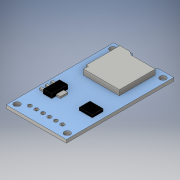
# Autodesk Inventor part: MicroSD Card Reader
Saved by Autodesk Inventor 2016 (Build 200138000, 138)
## iProperties
Created: 2015-11-27
Part Number: MicroSD Card Reader
Material: Generic
Document SubType Name: Modeling
Designer: Spooner
Density: 1 g/cm^3
Appearance: Default
Author: Spooner
Autodesk Inventor part; units mm, degrees
ref_plane "YZ Plane" through (0, 0, 0) normal (1, 0, 0) x (0, 1, 0)
ref_plane "XZ Plane" through (0, 0, 0) normal (0, 1, 0) x (-1, 0, 0)
ref_plane "XY Plane" through (0, 0, 0) normal (0, 0, 1) x (1, 0, 0)
sketch "Sketch1" plane through (0, 0, 0) normal (0, 1, 0) x (-1, 0, 0)
  line L0 (0, 0) -> (-23.5077, 0)
  line L1 (-23.5077, 0) -> (-23.5077, -41.9735)
  line L2 (0, -41.9735) -> (0, 0)
  line L3 (-7.4041, -41.9735) -> (-8.8011, -40.5765)
  line L4 (-8.8011, -40.5765) -> (-16.3322, -40.5765)
  line L5 (-16.3322, -40.5765) -> (-17.7292, -41.9735)
  line L6 (-23.5077, -41.9735) -> (-17.7292, -41.9735)
  line L7 (-7.4041, -41.9735) -> (0, -41.9735)
  circle A0 centre (-1.9431, -39.6748) radius 1.1811
  circle A1 centre (-21.5646, -39.6748) radius 1.1811
  circle A2 centre (-21.5646, -2.2987) radius 1.1811
  circle A3 centre (-1.9431, -2.2987) radius 1.1811
  dimension "d0" = 135
  dimension "d1" = 41.9735
  dimension "d2" = 23.5077
  dimension "d3" = 1.397
  dimension "d4" = 5.7785
  dimension "d5" = 7.4041
  dimension "d6" = 2.3622
  dimension "d7" = 1.1176
  dimension "d8" = 0.762
  dimension "d9" = 0.762
  dimension "d10" = 1.1176
  constraints: 16 end point, 4 centre point, 3 equal radius, 3 horizontal alignment, 3 parallel, 2 horizontal, 2 perpendicular, 2 vertical alignment
  measures "d0" angle of L4 L3
  measures "d1" distance of L2.start L0.start
  measures "d2" distance of L0.start L0.end
  measures "d3" distance between parallel lines of L4 L6
  measures "d4" distance of L1.end L5.end
  measures "d5" distance of L3.start L2.start
  measures "d6" diameter of A0
  measures "d7" distance edge to line of A1 L6
  measures "d8" distance edge to line of A1 L1
  measures "d9" distance edge to line of A0 L2
  measures "d10" distance edge to line of A2 L0
extrude "Extrusion1" add sketch "Sketch1" along normal blind 1.2446
sketch "Sketch2" plane through (0, 1.2446, 0) normal (0, 1, 0) x (1, 0, 0)
  line L0 (9.7028, 39.1795) -> (19.0627, 39.1795)
  line L1 (19.0627, 39.1795) -> (19.0627, 25.146)
  line L2 (19.0627, 25.146) -> (5.08, 25.146)
  line L3 (4.2418, 26.9875) -> (4.2418, 40.1955)
  line L4 (4.2418, 40.1955) -> (8.0518, 40.1955)
  line L5 (8.0518, 40.1955) -> (9.7028, 39.1795)
  line L6 (5.08, 25.146) -> (5.08, 26.9875)
  line L7 (16.3322, 40.5765) -> (8.8011, 40.5765) projected
  line L8 (0, 41.9735) -> (0, 0) projected
  line L9 (4.2418, 26.9875) -> (5.08, 26.9875)
  line L10 (7.4041, 41.9735) -> (0, 41.9735) projected
  point P0 (4.6609, 26.9875)
  dimension "d13" = 14.0335
  dimension "d14" = 1.397
  dimension "d15" = 14.8209
  dimension "d16" = 4.2418
  dimension "d17" = 5.08
  dimension "d18" = 13.208
  dimension "d20" = 1.778
  dimension "d21" = 9.3599
  dimension "d22" = 3.81
  constraints: 16 end point, 2 horizontal, 2 perpendicular, 1 horizontal alignment, 1 midpoint, 1 parallel, 1 vertical
  measures "d13" distance between parallel lines of L2 L0
  measures "d14" distance between parallel lines of L0 L7
  measures "d15" distance between parallel lines of L1 L3
  measures "d16" distance between parallel lines of L8 L3
  measures "d17" distance between parallel lines of L8 L6
  measures "d18" distance of L3.start L3.end
  measures "d20" distance between parallel lines of L4 L10
  measures "d21" distance from line of L0.start L1
  measures "d22" distance of L3.end L4.end
extrude "Extrusion2" add sketch "Sketch2" along normal blind 2.032
sketch "Sketch3" plane through (8.0518, 1.2446, -40.1955) normal (0, 0, -1) x (-1, 0, 0)
  line L0 (-10.1473, 1.778) -> (1.143, 1.778)
  line L1 (1.143, 1.778) -> (1.143, 1.0414)
  line L2 (1.143, 1.0414) -> (-10.1473, 1.0414)
  line L3 (-10.1473, 1.0414) -> (-10.1473, 1.778)
  line L4 (2.9718, 2.032) -> (-11.0109, 2.032) projected
  line L5 (-8.2804, -1.2446) -> (-0.7493, -1.2446) projected
  line L6 (-11.0109, 0) -> (-11.0109, 2.032) projected
  line L7 (3.81, 0) -> (3.81, 2.032) projected
  point P0 (8.0518, -1.2446)
  dimension "d25" = 0.254
  dimension "d26" = 2.286
  dimension "d27" = 0.8636
  dimension "d28" = 2.667
  constraints: 8 end point, 2 parallel, 1 horizontal, 1 perpendicular
  measures "d25" distance between parallel lines of L4 L0
  measures "d26" distance between parallel lines of L5 L2
  measures "d27" distance from line of L6 L0.start
  measures "d28" distance between parallel lines of L7 L1
extrude "Extrusion3" cut sketch "Sketch3" against normal blind 12.192
sketch "Sketch4" plane through (0, 1.2446, 0) normal (0, 1, 0) x (1, 0, 0)
  line L0 (3.5179, 10.9474) -> (6.8199, 10.9474)
  line L1 (6.8199, 10.9474) -> (6.8199, 17.3228)
  line L2 (6.8199, 17.3228) -> (3.5179, 17.3228)
  line L3 (3.5179, 17.3228) -> (3.5179, 10.9474)
  line L4 (5.08, 25.146) -> (19.0627, 25.146) projected
  line L5 (0, 41.9735) -> (0, 0) projected
  dimension "d31" = 6.3754
  dimension "d32" = 3.302
  dimension "d33" = 7.8232
  dimension "d34" = 3.5179
  constraints: 8 end point, 2 parallel, 1 horizontal, 1 perpendicular
  measures "d31" distance of L2.end L0.start
  measures "d32" distance of L1.end L2.end
  measures "d33" distance between parallel lines of L4 L2
  measures "d34" distance between parallel lines of L5 L3
extrude "Extrusion4" add sketch "Sketch4" along normal blind 1.6002
sketch "Sketch5" plane through (0, 1.2446, 0) normal (0, 1, 0) x (1, 0, 0)
  line L0 (3.5179, 10.9474) -> (3.5179, 17.3228) projected
  line L1 (1.4859, 16.764) -> (3.5179, 16.764)
  line L2 (3.5179, 16.764) -> (3.5179, 15.875)
  line L3 (3.5179, 15.875) -> (1.4859, 15.875)
  line L4 (1.4859, 15.875) -> (1.4859, 16.764)
  line L5 (1.4859, 14.5796) -> (3.5179, 14.5796)
  line L6 (3.5179, 14.5796) -> (3.5179, 13.6906)
  line L7 (3.5179, 13.6906) -> (1.4859, 13.6906)
  line L8 (1.4859, 13.6906) -> (1.4859, 14.5796)
  line L9 (1.4859, 12.3952) -> (3.5179, 12.3952)
  line L10 (3.5179, 12.3952) -> (3.5179, 11.5062)
  line L11 (3.5179, 11.5062) -> (1.4859, 11.5062)
  line L12 (1.4859, 11.5062) -> (1.4859, 12.3952)
  line L13 (3.5179, 17.3228) -> (3.5179, 10.9474) projected
  line L14 (6.8199, 17.3228) -> (6.8199, 10.9474) projected
  line L15 (6.8199, 15.5765) -> (8.4709, 15.5765)
  line L16 (8.4709, 15.5765) -> (8.4709, 12.6936)
  line L17 (8.4709, 12.6936) -> (6.8199, 12.6936)
  line L18 (6.8199, 12.6936) -> (6.8199, 15.5765)
  point P0 (0, 0)
  point P1 (1.4859, 14.1351)
  point P2 (3.5179, 14.1351)
  point P3 (8.4709, 14.1351)
  dimension "d37" = 0.889
  dimension "d38" = 2.032
  dimension "d39" = 5.2578
  dimension "d40" = 1.2954
  dimension "d41" = 1.2954
  dimension "d44" = 2.8829
  dimension "d45" = 1.651
  constraints: 32 end point, 8 parallel, 6 point on line, 4 horizontal, 4 perpendicular, 3 midpoint, 2 collinear, 2 horizontal alignment
  measures "d37" distance of L3.end L1.start
  measures "d38" distance of point (3.518, 14.135) point (1.486, 14.135)
  measures "d39" distance between parallel lines of L11 L1
  measures "d40" distance between parallel lines of L5 L3
  measures "d41" distance between parallel lines of L9 L7
  measures "d44" distance of L15.end L16.end
  measures "d45" distance from line of L14 point (8.471, 14.135)
extrude "Extrusion5" add sketch "Sketch5" along normal blind 0.635
sketch "Sketch6" plane through (0, 1.2446, 0) normal (0, 1, 0) x (1, 0, 0)
  line L0 (16.129, 16.637) -> (21.2598, 16.637)
  line L1 (21.2598, 16.637) -> (21.2598, 12.3698)
  line L2 (21.2598, 12.3698) -> (16.129, 12.3698)
  line L3 (16.129, 12.3698) -> (16.129, 16.637)
  line L4 (23.5077, 0) -> (23.5077, 41.9735) projected
  line L5 (5.08, 25.146) -> (19.0627, 25.146) projected
  point P0 (0, 0)
  dimension "d46" = 5.1308
  dimension "d47" = 4.2672
  dimension "d48" = 2.2479
  dimension "d49" = 8.509
  constraints: 8 end point, 2 parallel, 1 horizontal, 1 perpendicular
  measures "d46" distance of L0.start L0.end
  measures "d47" distance of L0.end L1.end
  measures "d48" distance between parallel lines of L4 L1
  measures "d49" distance between parallel lines of L5 L0
extrude "Extrusion6" add sketch "Sketch6" along normal blind 1.016
sketch "Sketch7" plane through (0, 1.2446, 0) normal (0, 1, 0) x (1, 0, 0)
  circle A0 centre (4.953, 4.318) radius 0.508
  line L0 (0, 0) -> (23.5077, 0) projected
  line L1 (0, 41.9735) -> (0, 0) projected
  dimension "d52" = 1.016
  dimension "d53" = 3.81
  dimension "d54" = 4.445
  constraints: 1 centre point
  measures "d52" diameter of A0
  measures "d53" distance edge to line of A0 L0
  measures "d54" distance edge to line of A0 L1
extrude "Extrusion7" cut sketch "Sketch7" against normal through all
sketch "Sketch8" plane through (0, 1.2446, 0) normal (0, 1, 0) x (1, 0, 0)
  circle A0 centre (4.953, 4.318) radius 0.762
  circle A1 centre (4.953, 4.318) radius 0.508 projected
  point P0 (0, 0)
  dimension "d57" = 1.524
  constraints: 1 centre point, 1 concentric
  measures "d57" diameter of A0
extrude "Extrusion8" add sketch "Sketch8" along normal blind 0.0254
pattern_linear "Rectangular Pattern1" count 6 spacing 2.54 along (1, 0, 0) of "Extrusion7", "Extrusion8"
sketch "Sketch9" plane through (0, 0, 0) normal (0, -1, 0) x (1, 0, 0)
  line L0 (18.4451, -5.588) -> (18.4451, -7.6539) construction
  line L1 (18.4451, -7.6539) -> (16.8609, -7.6539) construction
  line L2 (16.8609, -7.6539) -> (16.8609, -5.588) construction
  line L3 (16.8609, -5.588) -> (18.4451, -5.588) construction
  circle A0 centre (17.653, -4.318) radius 0.508 projected
  circle A1 centre (15.113, -4.318) radius 0.508 projected
  circle A2 centre (12.573, -4.318) radius 0.508 projected
  circle A3 centre (10.033, -4.318) radius 0.508 projected
  circle A4 centre (7.493, -4.318) radius 0.508 projected
  circle A5 centre (4.953, -4.318) radius 0.508 projected
  line L4 (13.825, -5.588) -> (13.825, -7.6539) construction
  line L5 (13.825, -7.6539) -> (16.401, -7.6539) construction
  line L6 (16.401, -7.6539) -> (16.401, -5.588) construction
  line L7 (16.401, -5.588) -> (13.825, -5.588) construction
  line L8 (13.5877, -5.588) -> (13.5877, -7.6539) construction
  line L9 (13.5877, -7.6539) -> (11.5583, -7.6539) construction
  line L10 (11.5583, -7.6539) -> (11.5583, -5.588) construction
  line L11 (11.5583, -5.588) -> (13.5877, -5.588) construction
  line L12 (10.3041, -5.588) -> (10.3041, -7.6539) construction
  line L13 (10.3041, -7.6539) -> (9.7619, -7.6539) construction
  line L14 (9.7619, -7.6539) -> (9.7619, -5.588) construction
  line L15 (9.7619, -5.588) -> (10.3041, -5.588) construction
  line L16 (7.9729, -5.588) -> (7.9729, -7.6539) construction
  line L17 (7.9729, -7.6539) -> (7.0131, -7.6539) construction
  line L18 (7.0131, -7.6539) -> (7.0131, -5.588) construction
  line L19 (7.0131, -5.588) -> (7.9729, -5.588) construction
  line L20 (5.7817, -5.588) -> (5.7817, -7.6539) construction
  line L21 (5.7817, -7.6539) -> (4.1243, -7.6539) construction
  line L22 (4.1243, -7.6539) -> (4.1243, -5.588) construction
  line L23 (4.1243, -5.588) -> (5.7817, -5.588) construction
  spline S0 degree 2 poles (17.2026, -6.5593) (17.0886, -6.4666) (17.0006, -6.2897) (17.0006, -6.165) knots 0 0 0 1 2 2 2
  spline S1 degree 2 poles (17.0006, -6.165) (17.0006, -5.9524) (17.1804, -5.818) knots 0 0 0 1 1 1
  spline S2 degree 2 poles (17.1804, -5.818) (17.3621, -5.6798) (17.6559, -5.6798) knots 0 0 0 1 1 1
  spline S3 degree 2 poles (17.6559, -5.6798) (17.9806, -5.6798) (18.1508, -5.8354) knots 0 0 0 1 1 1
  spline S4 degree 2 poles (18.1508, -5.8354) (18.287, -5.9601) (18.287, -6.1399) knots 0 0 0 1 1 1
  spline S5 degree 2 poles (18.287, -6.1399) (18.287, -6.28) (18.2455, -6.3612) knots 0 0 0 1 1 1
  spline S6 degree 2 poles (18.2455, -6.3612) (18.1991, -6.4511) (18.0841, -6.5139) knots 0 0 0 1 1 1
  spline S7 degree 2 poles (18.0841, -6.5139) (18.0599, -6.5275) (18.0377, -6.5275) knots 0 0 0 1 1 1
  spline S8 degree 2 poles (18.0377, -6.5275) (17.999, -6.5275) (17.9459, -6.4695) (17.9459, -6.4337) knots 0 0 0 1 2 2 2
  spline S9 degree 2 poles (17.9459, -6.4337) (17.9459, -6.3834) (18, -6.3544) knots 0 0 0 1 1 1
  spline S10 degree 2 poles (18, -6.3544) (18.056, -6.3216) (18.0802, -6.2655) knots 0 0 0 1 1 1
  spline S11 degree 2 poles (18.0802, -6.2655) (18.1005, -6.223) (18.1005, -6.1389) knots 0 0 0 1 1 1
  spline S12 degree 2 poles (18.1005, -6.1389) (18.1005, -6.0297) (18.0029, -5.9543) knots 0 0 0 1 1 1
  spline S13 degree 2 poles (18.0029, -5.9543) (17.885, -5.8615) (17.6559, -5.8615) knots 0 0 0 1 1 1
  spline S14 degree 2 poles (17.6559, -5.8615) (17.4452, -5.8615) (17.1871, -6.0365) (17.1871, -6.1679) knots 0 0 0 1 2 2 2
  spline S15 degree 2 poles (17.1871, -6.1679) (17.1871, -6.31) (17.3225, -6.4173) knots 0 0 0 1 1 1
  spline S16 degree 2 poles (17.3225, -6.4173) (17.3553, -6.4443) (17.3553, -6.4859) knots 0 0 0 1 1 1
  spline S17 degree 2 poles (17.3553, -6.4859) (17.3553, -6.5217) (17.2983, -6.5816) (17.2606, -6.5816) knots 0 0 0 1 2 2 2
  spline S18 degree 2 poles (17.2606, -6.5816) (17.2297, -6.5816) (17.2026, -6.5593) knots 0 0 0 1 1 1
  spline S19 degree 2 poles (17.3669, -7.6718) (17.0006, -7.6718) (17.0006, -7.2195) knots 0 0 0 1 1 1
  spline S20 degree 2 poles (17.0006, -7.2195) (17.0006, -6.9479) (17.2722, -6.801) knots 0 0 0 1 1 1
  spline S21 degree 2 poles (17.2722, -6.801) (17.2896, -6.7903) (17.3167, -6.7903) knots 0 0 0 1 1 1
  spline S22 degree 2 poles (17.3167, -6.7903) (17.3572, -6.7903) (17.4201, -6.8503) (17.4201, -6.8889) knots 0 0 0 1 2 2 2
  spline S23 degree 2 poles (17.4201, -6.8889) (17.4201, -6.9353) (17.3775, -6.9537) knots 0 0 0 1 1 1
  spline S24 degree 2 poles (17.3775, -6.9537) (17.1871, -7.0397) (17.1871, -7.2195) knots 0 0 0 1 1 1
  spline S25 degree 2 poles (17.1871, -7.2195) (17.1871, -7.4843) (17.365, -7.4843) knots 0 0 0 1 1 1
  spline S26 degree 2 poles (17.365, -7.4843) (17.4529, -7.4843) (17.5225, -7.3181) knots 0 0 0 1 1 1
  spline S27 degree 2 poles (17.5225, -7.3181) (17.6569, -6.9972) (17.6598, -6.9904) knots 0 0 0 1 1 1
  spline S28 degree 2 poles (17.6598, -6.9904) (17.7728, -6.801) (17.9594, -6.801) knots 0 0 0 1 1 1
  spline S29 degree 2 poles (17.9594, -6.801) (18.1334, -6.801) (18.2232, -6.9286) knots 0 0 0 1 1 1
  spline S30 degree 2 poles (18.2232, -6.9286) (18.2938, -7.03) (18.2996, -7.1934) knots 0 0 0 1 1 1
  spline S31 degree 2 poles (18.2996, -7.1934) (18.3054, -7.3442) (18.2271, -7.4659) knots 0 0 0 1 1 1
  spline S32 degree 2 poles (18.2271, -7.4659) (18.1633, -7.5781) (18.0319, -7.6196) knots 0 0 0 1 1 1
  spline S33 degree 2 poles (18.0319, -7.6196) (18.0106, -7.6254) (17.9961, -7.6254) knots 0 0 0 1 1 1
  spline S34 degree 2 poles (17.9961, -7.6254) (17.9575, -7.6254) (17.9101, -7.5684) (17.9101, -7.5317) knots 0 0 0 1 2 2 2
  spline S35 degree 2 poles (17.9101, -7.5317) (17.9101, -7.464) (17.9623, -7.4476) knots 0 0 0 1 1 1
  spline S36 degree 2 poles (17.9623, -7.4476) (18.0415, -7.4224) (18.1208, -7.2842) (18.1169, -7.2001) knots 0 0 0 1 2 2 2
  spline S37 degree 2 poles (18.1169, -7.2001) (18.1082, -6.9827) (17.9633, -6.9827) knots 0 0 0 1 1 1
  spline S38 degree 2 poles (17.9633, -6.9827) (17.8869, -6.9827) (17.8337, -7.059) knots 0 0 0 1 1 1
  spline S39 degree 2 poles (17.8337, -7.059) (17.7931, -7.1161) (17.7439, -7.2523) knots 0 0 0 1 1 1
  spline S40 degree 2 poles (17.7439, -7.2523) (17.6694, -7.4592) (17.6201, -7.5307) knots 0 0 0 1 1 1
  spline S41 degree 2 poles (17.6201, -7.5307) (17.5225, -7.6718) (17.3669, -7.6718) knots 0 0 0 1 1 1
  spline S42 degree 2 poles (14.8269, -6.5439) (14.4606, -6.5439) (14.4606, -6.0916) knots 0 0 0 1 1 1
  spline S43 degree 2 poles (14.4606, -6.0916) (14.4606, -5.82) (14.7322, -5.6731) knots 0 0 0 1 1 1
  spline S44 degree 2 poles (14.7322, -5.6731) (14.7496, -5.6624) (14.7767, -5.6624) knots 0 0 0 1 1 1
  spline S45 degree 2 poles (14.7767, -5.6624) (14.8172, -5.6624) (14.8801, -5.7223) (14.8801, -5.761) knots 0 0 0 1 2 2 2
  spline S46 degree 2 poles (14.8801, -5.761) (14.8801, -5.8074) (14.8375, -5.8258) knots 0 0 0 1 1 1
  spline S47 degree 2 poles (14.8375, -5.8258) (14.6471, -5.9118) (14.6471, -6.0916) knots 0 0 0 1 1 1
  spline S48 degree 2 poles (14.6471, -6.0916) (14.6471, -6.3564) (14.825, -6.3564) knots 0 0 0 1 1 1
  spline S49 degree 2 poles (14.825, -6.3564) (14.9129, -6.3564) (14.9825, -6.1901) knots 0 0 0 1 1 1
  spline S50 degree 2 poles (14.9825, -6.1901) (15.1169, -5.8693) (15.1198, -5.8625) knots 0 0 0 1 1 1
  spline S51 degree 2 poles (15.1198, -5.8625) (15.2328, -5.6731) (15.4194, -5.6731) knots 0 0 0 1 1 1
  spline S52 degree 2 poles (15.4194, -5.6731) (15.5934, -5.6731) (15.6832, -5.8006) knots 0 0 0 1 1 1
  spline S53 degree 2 poles (15.6832, -5.8006) (15.7538, -5.9021) (15.7596, -6.0655) knots 0 0 0 1 1 1
  spline S54 degree 2 poles (15.7596, -6.0655) (15.7654, -6.2162) (15.6871, -6.338) knots 0 0 0 1 1 1
  spline S55 degree 2 poles (15.6871, -6.338) (15.6233, -6.4501) (15.4919, -6.4917) knots 0 0 0 1 1 1
  spline S56 degree 2 poles (15.4919, -6.4917) (15.4706, -6.4975) (15.4561, -6.4975) knots 0 0 0 1 1 1
  spline S57 degree 2 poles (15.4561, -6.4975) (15.4175, -6.4975) (15.3701, -6.4405) (15.3701, -6.4037) knots 0 0 0 1 2 2 2
  spline S58 degree 2 poles (15.3701, -6.4037) (15.3701, -6.3361) (15.4223, -6.3197) knots 0 0 0 1 1 1
  spline S59 degree 2 poles (15.4223, -6.3197) (15.5015, -6.2945) (15.5808, -6.1563) (15.5769, -6.0722) knots 0 0 0 1 2 2 2
  spline S60 degree 2 poles (15.5769, -6.0722) (15.5682, -5.8548) (15.4233, -5.8548) knots 0 0 0 1 1 1
  spline S61 degree 2 poles (15.4233, -5.8548) (15.3469, -5.8548) (15.2937, -5.9311) knots 0 0 0 1 1 1
  spline S62 degree 2 poles (15.2937, -5.9311) (15.2531, -5.9881) (15.2039, -6.1244) knots 0 0 0 1 1 1
  spline S63 degree 2 poles (15.2039, -6.1244) (15.1294, -6.3312) (15.0801, -6.4028) knots 0 0 0 1 1 1
  spline S64 degree 2 poles (15.0801, -6.4028) (14.9825, -6.5439) (14.8269, -6.5439) knots 0 0 0 1 1 1
  spline S65 degree 2 poles (14.6626, -7.6196) (14.5486, -7.5268) (14.4606, -7.35) (14.4606, -7.2253) knots 0 0 0 1 2 2 2
  spline S66 degree 2 poles (14.4606, -7.2253) (14.4606, -7.0126) (14.6404, -6.8783) knots 0 0 0 1 1 1
  spline S67 degree 2 poles (14.6404, -6.8783) (14.8221, -6.7401) (15.1159, -6.7401) knots 0 0 0 1 1 1
  spline S68 degree 2 poles (15.1159, -6.7401) (15.4406, -6.7401) (15.6108, -6.8957) knots 0 0 0 1 1 1
  spline S69 degree 2 poles (15.6108, -6.8957) (15.747, -7.0204) (15.747, -7.2001) knots 0 0 0 1 1 1
  spline S70 degree 2 poles (15.747, -7.2001) (15.747, -7.3403) (15.7055, -7.4215) knots 0 0 0 1 1 1
  spline S71 degree 2 poles (15.7055, -7.4215) (15.6591, -7.5114) (15.5441, -7.5742) knots 0 0 0 1 1 1
  spline S72 degree 2 poles (15.5441, -7.5742) (15.5199, -7.5877) (15.4977, -7.5877) knots 0 0 0 1 1 1
  spline S73 degree 2 poles (15.4977, -7.5877) (15.459, -7.5877) (15.4059, -7.5297) (15.4059, -7.494) knots 0 0 0 1 2 2 2
  spline S74 degree 2 poles (15.4059, -7.494) (15.4059, -7.4437) (15.46, -7.4147) knots 0 0 0 1 1 1
  spline S75 degree 2 poles (15.46, -7.4147) (15.516, -7.3819) (15.5402, -7.3258) knots 0 0 0 1 1 1
  spline S76 degree 2 poles (15.5402, -7.3258) (15.5605, -7.2833) (15.5605, -7.1992) knots 0 0 0 1 1 1
  spline S77 degree 2 poles (15.5605, -7.1992) (15.5605, -7.09) (15.4629, -7.0146) knots 0 0 0 1 1 1
  spline S78 degree 2 poles (15.4629, -7.0146) (15.345, -6.9218) (15.1159, -6.9218) knots 0 0 0 1 1 1
  spline S79 degree 2 poles (15.1159, -6.9218) (14.9052, -6.9218) (14.6471, -7.0967) (14.6471, -7.2282) knots 0 0 0 1 2 2 2
  spline S80 degree 2 poles (14.6471, -7.2282) (14.6471, -7.3703) (14.7825, -7.4775) knots 0 0 0 1 1 1
  spline S81 degree 2 poles (14.7825, -7.4775) (14.8153, -7.5046) (14.8153, -7.5462) knots 0 0 0 1 1 1
  spline S82 degree 2 poles (14.8153, -7.5462) (14.8153, -7.5819) (14.7583, -7.6418) (14.7206, -7.6418) knots 0 0 0 1 2 2 2
  spline S83 degree 2 poles (14.7206, -7.6418) (14.6897, -7.6418) (14.6626, -7.6196) knots 0 0 0 1 1 1
  spline S84 degree 2 poles (14.5969, -8.7253) (14.5882, -8.7359) (14.565, -8.7359) knots 0 0 0 1 1 1
  spline S85 degree 2 poles (14.565, -8.7359) (14.5263, -8.7359) (14.4712, -8.676) (14.4712, -8.6403) knots 0 0 0 1 2 2 2
  spline S86 degree 2 poles (14.4712, -8.6403) (14.4712, -8.5919) (14.5215, -8.5629) knots 0 0 0 1 1 1
  line L24 (14.5215, -8.5629) -> (15.1903, -8.1879)
  line L25 (15.1903, -8.1879) -> (15.0473, -8.0555)
  line L26 (15.0473, -8.0555) -> (14.565, -8.0555)
  spline S87 degree 2 poles (14.565, -8.0555) (14.4712, -8.0555) (14.4712, -7.9656) knots 0 0 0 1 1 1
  spline S88 degree 2 poles (14.4712, -7.9656) (14.4712, -7.8738) (14.565, -7.8738) knots 0 0 0 1 1 1
  line L27 (14.565, -7.8738) -> (15.6417, -7.8738)
  spline S89 degree 2 poles (15.6417, -7.8738) (15.7345, -7.8738) (15.7345, -7.9656) knots 0 0 0 1 1 1
  spline S90 degree 2 poles (15.7345, -7.9656) (15.7345, -8.0555) (15.6417, -8.0555) knots 0 0 0 1 1 1
  line L28 (15.6417, -8.0555) -> (15.2744, -8.0555)
  line L29 (15.2744, -8.0555) -> (15.7074, -8.4924)
  spline S91 degree 2 poles (15.7074, -8.4924) (15.7345, -8.5194) (15.7345, -8.5542) knots 0 0 0 1 1 1
  spline S92 degree 2 poles (15.7345, -8.5542) (15.7345, -8.591) (15.6765, -8.6461) (15.6407, -8.6461) knots 0 0 0 1 2 2 2
  spline S93 degree 2 poles (15.6407, -8.6461) (15.6021, -8.6461) (15.5905, -8.62) knots 0 0 0 1 1 1
  line L30 (15.5905, -8.62) -> (15.3073, -8.3145)
  line L31 (15.3073, -8.3145) -> (14.5969, -8.7253)
  spline S94 degree 2 poles (12.0231, -6.7198) (11.9293, -6.7198) (11.9293, -6.628) knots 0 0 0 1 1 1
  spline S95 degree 2 poles (11.9293, -6.628) (11.9293, -6.5362) (12.0231, -6.5362) knots 0 0 0 1 1 1
  line L32 (12.0231, -6.5362) -> (12.8765, -6.5362)
  line L33 (12.8765, -6.5362) -> (12.4947, -6.3023)
  spline S96 degree 2 poles (12.4947, -6.3023) (12.4358, -6.2607) (12.4358, -6.2008) knots 0 0 0 1 1 1
  spline S97 degree 2 poles (12.4358, -6.2008) (12.4358, -6.1428) (12.4899, -6.107) knots 0 0 0 1 1 1
  line L34 (12.4899, -6.107) -> (12.8852, -5.8751)
  line L35 (12.8852, -5.8751) -> (12.0231, -5.8751)
  spline S98 degree 2 poles (12.0231, -5.8751) (11.9293, -5.8751) (11.9293, -5.7832) knots 0 0 0 1 1 1
  spline S99 degree 2 poles (11.9293, -5.7832) (11.9293, -5.6895) (12.0231, -5.6895) knots 0 0 0 1 1 1
  line L36 (12.0231, -5.6895) -> (13.092, -5.6895)
  spline S100 degree 2 poles (13.092, -5.6895) (13.1906, -5.6895) (13.1906, -5.789) knots 0 0 0 1 1 1
  spline S101 degree 2 poles (13.1906, -5.789) (13.1906, -5.8577) (13.1355, -5.8963) knots 0 0 0 1 1 1
  line L37 (13.1355, -5.8963) -> (12.6774, -6.2037)
  line L38 (12.6774, -6.2037) -> (13.1258, -6.5072)
  spline S102 degree 2 poles (13.1258, -6.5072) (13.1993, -6.5584) (13.1993, -6.6241) knots 0 0 0 1 1 1
  spline S103 degree 2 poles (13.1993, -6.6241) (13.1993, -6.6647) (13.1374, -6.7198) (13.092, -6.7198) knots 0 0 0 1 2 2 2
  line L39 (13.092, -6.7198) -> (12.0231, -6.7198)
  spline S104 degree 2 poles (12.5585, -7.9511) (12.3033, -7.9511) (12.1371, -7.8313) knots 0 0 0 1 1 1
  spline S105 degree 2 poles (12.1371, -7.8313) (11.9206, -7.6911) (11.9206, -7.4756) knots 0 0 0 1 1 1
  spline S106 degree 2 poles (11.9206, -7.4756) (11.9206, -7.2591) (12.1207, -7.1209) knots 0 0 0 1 1 1
  spline S107 degree 2 poles (12.1207, -7.1209) (12.3043, -6.9923) (12.5585, -6.9923) knots 0 0 0 1 1 1
  spline S108 degree 2 poles (12.5585, -6.9923) (12.8127, -6.9923) (12.9992, -7.1132) knots 0 0 0 1 1 1
  spline S109 degree 2 poles (12.9992, -7.1132) (13.207, -7.2465) (13.207, -7.4553) knots 0 0 0 1 1 1
  spline S110 degree 2 poles (13.207, -7.4553) (13.207, -7.6786) (13.0002, -7.8226) knots 0 0 0 1 1 1
  spline S111 degree 2 poles (13.0002, -7.8226) (12.8127, -7.9511) (12.5585, -7.9511) knots 0 0 0 1 1 1
  spline S112 degree 2 poles (12.5585, -7.7675) (12.7441, -7.7675) (12.8833, -7.6863) knots 0 0 0 1 1 1
  spline S113 degree 2 poles (12.8833, -7.6863) (13.0205, -7.6012) (13.0205, -7.4553) knots 0 0 0 1 1 1
  spline S114 degree 2 poles (13.0205, -7.4553) (13.0205, -7.321) (12.8678, -7.2378) knots 0 0 0 1 1 1
  spline S115 degree 2 poles (12.8678, -7.2378) (12.7489, -7.176) (12.5585, -7.176) knots 0 0 0 1 1 1
  spline S116 degree 2 poles (12.5585, -7.176) (12.372, -7.176) (12.255, -7.233) knots 0 0 0 1 1 1
  spline S117 degree 2 poles (12.255, -7.233) (12.1071, -7.3345) (12.1071, -7.4756) knots 0 0 0 1 1 1
  spline S118 degree 2 poles (12.1071, -7.4756) (12.1071, -7.6148) (12.255, -7.7018) knots 0 0 0 1 1 1
  spline S119 degree 2 poles (12.255, -7.7018) (12.37, -7.7675) (12.5585, -7.7675) knots 0 0 0 1 1 1
  spline S120 degree 2 poles (12.2869, -9.0201) (11.9206, -9.0201) (11.9206, -8.5678) knots 0 0 0 1 1 1
  spline S121 degree 2 poles (11.9206, -8.5678) (11.9206, -8.2962) (12.1922, -8.1493) knots 0 0 0 1 1 1
  spline S122 degree 2 poles (12.1922, -8.1493) (12.2096, -8.1386) (12.2367, -8.1386) knots 0 0 0 1 1 1
  spline S123 degree 2 poles (12.2367, -8.1386) (12.2772, -8.1386) (12.3401, -8.1986) (12.3401, -8.2372) knots 0 0 0 1 2 2 2
  spline S124 degree 2 poles (12.3401, -8.2372) (12.3401, -8.2836) (12.2975, -8.302) knots 0 0 0 1 1 1
  spline S125 degree 2 poles (12.2975, -8.302) (12.1071, -8.388) (12.1071, -8.5678) knots 0 0 0 1 1 1
  spline S126 degree 2 poles (12.1071, -8.5678) (12.1071, -8.8326) (12.285, -8.8326) knots 0 0 0 1 1 1
  spline S127 degree 2 poles (12.285, -8.8326) (12.3729, -8.8326) (12.4425, -8.6663) knots 0 0 0 1 1 1
  spline S128 degree 2 poles (12.4425, -8.6663) (12.5769, -8.3455) (12.5798, -8.3387) knots 0 0 0 1 1 1
  spline S129 degree 2 poles (12.5798, -8.3387) (12.6928, -8.1493) (12.8794, -8.1493) knots 0 0 0 1 1 1
  spline S130 degree 2 poles (12.8794, -8.1493) (13.0534, -8.1493) (13.1432, -8.2768) knots 0 0 0 1 1 1
  spline S131 degree 2 poles (13.1432, -8.2768) (13.2138, -8.3783) (13.2196, -8.5417) knots 0 0 0 1 1 1
  spline S132 degree 2 poles (13.2196, -8.5417) (13.2254, -8.6924) (13.1471, -8.8142) knots 0 0 0 1 1 1
  spline S133 degree 2 poles (13.1471, -8.8142) (13.0833, -8.9263) (12.9519, -8.9679) knots 0 0 0 1 1 1
  spline S134 degree 2 poles (12.9519, -8.9679) (12.9306, -8.9737) (12.9161, -8.9737) knots 0 0 0 1 1 1
  spline S135 degree 2 poles (12.9161, -8.9737) (12.8775, -8.9737) (12.8301, -8.9167) (12.8301, -8.8799) knots 0 0 0 1 2 2 2
  spline S136 degree 2 poles (12.8301, -8.8799) (12.8301, -8.8123) (12.8823, -8.7959) knots 0 0 0 1 1 1
  spline S137 degree 2 poles (12.8823, -8.7959) (12.9615, -8.7707) (13.0408, -8.6325) (13.0369, -8.5484) knots 0 0 0 1 2 2 2
  spline S138 degree 2 poles (13.0369, -8.5484) (13.0282, -8.331) (12.8833, -8.331) knots 0 0 0 1 1 1
  spline S139 degree 2 poles (12.8833, -8.331) (12.8069, -8.331) (12.7537, -8.4073) knots 0 0 0 1 1 1
  spline S140 degree 2 poles (12.7537, -8.4073) (12.7131, -8.4643) (12.6639, -8.6006) knots 0 0 0 1 1 1
  spline S141 degree 2 poles (12.6639, -8.6006) (12.5894, -8.8075) (12.5401, -8.879) knots 0 0 0 1 1 1
  spline S142 degree 2 poles (12.5401, -8.879) (12.4425, -9.0201) (12.2869, -9.0201) knots 0 0 0 1 1 1
  spline S143 degree 2 poles (12.025, -9.4473) (11.9293, -9.4473) (11.9293, -9.3555) knots 0 0 0 1 1 1
  spline S144 degree 2 poles (11.9293, -9.3555) (11.9293, -9.2637) (12.025, -9.2637) knots 0 0 0 1 1 1
  line L40 (12.025, -9.2637) -> (13.1026, -9.2637)
  spline S145 degree 2 poles (13.1026, -9.2637) (13.1954, -9.2637) (13.1954, -9.3555) knots 0 0 0 1 1 1
  spline S146 degree 2 poles (13.1954, -9.3555) (13.1954, -9.4473) (13.1026, -9.4473) knots 0 0 0 1 1 1
  line L41 (13.1026, -9.4473) -> (12.025, -9.4473)
  spline S147 degree 2 poles (9.4831, -6.7198) (9.3893, -6.7198) (9.3893, -6.628) knots 0 0 0 1 1 1
  spline S148 degree 2 poles (9.3893, -6.628) (9.3893, -6.5362) (9.4831, -6.5362) knots 0 0 0 1 1 1
  line L42 (9.4831, -6.5362) -> (10.3365, -6.5362)
  line L43 (10.3365, -6.5362) -> (9.9547, -6.3023)
  spline S149 degree 2 poles (9.9547, -6.3023) (9.8958, -6.2607) (9.8958, -6.2008) knots 0 0 0 1 1 1
  spline S150 degree 2 poles (9.8958, -6.2008) (9.8958, -6.1428) (9.9499, -6.107) knots 0 0 0 1 1 1
  line L44 (9.9499, -6.107) -> (10.3452, -5.8751)
  line L45 (10.3452, -5.8751) -> (9.4831, -5.8751)
  spline S151 degree 2 poles (9.4831, -5.8751) (9.3893, -5.8751) (9.3893, -5.7832) knots 0 0 0 1 1 1
  spline S152 degree 2 poles (9.3893, -5.7832) (9.3893, -5.6895) (9.4831, -5.6895) knots 0 0 0 1 1 1
  line L46 (9.4831, -5.6895) -> (10.552, -5.6895)
  spline S153 degree 2 poles (10.552, -5.6895) (10.6506, -5.6895) (10.6506, -5.789) knots 0 0 0 1 1 1
  spline S154 degree 2 poles (10.6506, -5.789) (10.6506, -5.8577) (10.5955, -5.8963) knots 0 0 0 1 1 1
  line L47 (10.5955, -5.8963) -> (10.1374, -6.2037)
  line L48 (10.1374, -6.2037) -> (10.5858, -6.5072)
  spline S155 degree 2 poles (10.5858, -6.5072) (10.6593, -6.5584) (10.6593, -6.6241) knots 0 0 0 1 1 1
  spline S156 degree 2 poles (10.6593, -6.6241) (10.6593, -6.6647) (10.5974, -6.7198) (10.552, -6.7198) knots 0 0 0 1 2 2 2
  line L49 (10.552, -6.7198) -> (9.4831, -6.7198)
  spline S157 degree 2 poles (9.485, -7.2175) (9.3893, -7.2175) (9.3893, -7.1257) knots 0 0 0 1 1 1
  spline S158 degree 2 poles (9.3893, -7.1257) (9.3893, -7.0339) (9.485, -7.0339) knots 0 0 0 1 1 1
  line L50 (9.485, -7.0339) -> (10.5626, -7.0339)
  spline S159 degree 2 poles (10.5626, -7.0339) (10.6554, -7.0339) (10.6554, -7.1257) knots 0 0 0 1 1 1
  spline S160 degree 2 poles (10.6554, -7.1257) (10.6554, -7.2175) (10.5626, -7.2175) knots 0 0 0 1 1 1
  line L51 (10.5626, -7.2175) -> (9.485, -7.2175)
  spline S161 degree 2 poles (9.7469, -8.4006) (9.3806, -8.4006) (9.3806, -7.9482) knots 0 0 0 1 1 1
  spline S162 degree 2 poles (9.3806, -7.9482) (9.3806, -7.6766) (9.6522, -7.5297) knots 0 0 0 1 1 1
  spline S163 degree 2 poles (9.6522, -7.5297) (9.6696, -7.5191) (9.6967, -7.5191) knots 0 0 0 1 1 1
  spline S164 degree 2 poles (9.6967, -7.5191) (9.7372, -7.5191) (9.8001, -7.579) (9.8001, -7.6177) knots 0 0 0 1 2 2 2
  spline S165 degree 2 poles (9.8001, -7.6177) (9.8001, -7.6641) (9.7575, -7.6824) knots 0 0 0 1 1 1
  spline S166 degree 2 poles (9.7575, -7.6824) (9.5671, -7.7685) (9.5671, -7.9482) knots 0 0 0 1 1 1
  spline S167 degree 2 poles (9.5671, -7.9482) (9.5671, -8.2131) (9.745, -8.2131) knots 0 0 0 1 1 1
  spline S168 degree 2 poles (9.745, -8.2131) (9.8329, -8.2131) (9.9025, -8.0468) knots 0 0 0 1 1 1
  spline S169 degree 2 poles (9.9025, -8.0468) (10.0369, -7.7259) (10.0398, -7.7192) knots 0 0 0 1 1 1
  spline S170 degree 2 poles (10.0398, -7.7192) (10.1528, -7.5297) (10.3394, -7.5297) knots 0 0 0 1 1 1
  spline S171 degree 2 poles (10.3394, -7.5297) (10.5134, -7.5297) (10.6032, -7.6573) knots 0 0 0 1 1 1
  spline S172 degree 2 poles (10.6032, -7.6573) (10.6738, -7.7588) (10.6796, -7.9221) knots 0 0 0 1 1 1
  spline S173 degree 2 poles (10.6796, -7.9221) (10.6854, -8.0729) (10.6071, -8.1947) knots 0 0 0 1 1 1
  spline S174 degree 2 poles (10.6071, -8.1947) (10.5433, -8.3068) (10.4119, -8.3484) knots 0 0 0 1 1 1
  spline S175 degree 2 poles (10.4119, -8.3484) (10.3906, -8.3542) (10.3761, -8.3542) knots 0 0 0 1 1 1
  spline S176 degree 2 poles (10.3761, -8.3542) (10.3375, -8.3542) (10.2901, -8.2971) (10.2901, -8.2604) knots 0 0 0 1 2 2 2
  spline S177 degree 2 poles (10.2901, -8.2604) (10.2901, -8.1928) (10.3423, -8.1763) knots 0 0 0 1 1 1
  spline S178 degree 2 poles (10.3423, -8.1763) (10.4215, -8.1512) (10.5008, -8.013) (10.4969, -7.9289) knots 0 0 0 1 2 2 2
  spline S179 degree 2 poles (10.4969, -7.9289) (10.4882, -7.7114) (10.3433, -7.7114) knots 0 0 0 1 1 1
  spline S180 degree 2 poles (10.3433, -7.7114) (10.2669, -7.7114) (10.2137, -7.7878) knots 0 0 0 1 1 1
  spline S181 degree 2 poles (10.2137, -7.7878) (10.1731, -7.8448) (10.1239, -7.9811) knots 0 0 0 1 1 1
  spline S182 degree 2 poles (10.1239, -7.9811) (10.0494, -8.1879) (10.0001, -8.2594) knots 0 0 0 1 1 1
  spline S183 degree 2 poles (10.0001, -8.2594) (9.9025, -8.4006) (9.7469, -8.4006) knots 0 0 0 1 1 1
  spline S184 degree 2 poles (10.0185, -9.5613) (9.7633, -9.5613) (9.5971, -9.4415) knots 0 0 0 1 1 1
  spline S185 degree 2 poles (9.5971, -9.4415) (9.3806, -9.3013) (9.3806, -9.0858) knots 0 0 0 1 1 1
  spline S186 degree 2 poles (9.3806, -9.0858) (9.3806, -8.8693) (9.5807, -8.7311) knots 0 0 0 1 1 1
  spline S187 degree 2 poles (9.5807, -8.7311) (9.7643, -8.6026) (10.0185, -8.6026) knots 0 0 0 1 1 1
  spline S188 degree 2 poles (10.0185, -8.6026) (10.2727, -8.6026) (10.4592, -8.7234) knots 0 0 0 1 1 1
  spline S189 degree 2 poles (10.4592, -8.7234) (10.667, -8.8568) (10.667, -9.0655) knots 0 0 0 1 1 1
  spline S190 degree 2 poles (10.667, -9.0655) (10.667, -9.2888) (10.4602, -9.4328) knots 0 0 0 1 1 1
  spline S191 degree 2 poles (10.4602, -9.4328) (10.2727, -9.5613) (10.0185, -9.5613) knots 0 0 0 1 1 1
  spline S192 degree 2 poles (10.0185, -9.3777) (10.2041, -9.3777) (10.3433, -9.2965) knots 0 0 0 1 1 1
  spline S193 degree 2 poles (10.3433, -9.2965) (10.4805, -9.2115) (10.4805, -9.0655) knots 0 0 0 1 1 1
  spline S194 degree 2 poles (10.4805, -9.0655) (10.4805, -8.9312) (10.3278, -8.8481) knots 0 0 0 1 1 1
  spline S195 degree 2 poles (10.3278, -8.8481) (10.2089, -8.7862) (10.0185, -8.7862) knots 0 0 0 1 1 1
  spline S196 degree 2 poles (10.0185, -8.7862) (9.832, -8.7862) (9.715, -8.8432) knots 0 0 0 1 1 1
  spline S197 degree 2 poles (9.715, -8.8432) (9.5671, -8.9447) (9.5671, -9.0858) knots 0 0 0 1 1 1
  spline S198 degree 2 poles (9.5671, -9.0858) (9.5671, -9.225) (9.715, -9.312) knots 0 0 0 1 1 1
  spline S199 degree 2 poles (9.715, -9.312) (9.83, -9.3777) (10.0185, -9.3777) knots 0 0 0 1 1 1
  line L52 (8.0096, -6.5323) -> (6.9329, -6.2288)
  spline S200 degree 2 poles (6.9329, -6.2288) (6.8546, -6.2075) (6.8546, -6.1167) knots 0 0 0 1 1 1
  spline S201 degree 2 poles (6.8546, -6.1167) (6.8546, -6.0249) (6.93, -6.0017) knots 0 0 0 1 1 1
  line L53 (6.93, -6.0017) -> (8.0048, -5.6605)
  spline S202 degree 2 poles (8.0048, -5.6605) (8.0212, -5.6566) (8.0376, -5.6566) knots 0 0 0 1 1 1
  spline S203 degree 2 poles (8.0376, -5.6566) (8.0753, -5.6566) (8.1266, -5.7127) (8.1266, -5.7504) knots 0 0 0 1 2 2 2
  spline S204 degree 2 poles (8.1266, -5.7504) (8.1266, -5.8142) (8.0396, -5.8354) knots 0 0 0 1 1 1
  line L54 (8.0396, -5.8354) -> (7.1552, -6.1148)
  line L55 (7.1552, -6.1148) -> (8.0647, -6.3583)
  spline S205 degree 2 poles (8.0647, -6.3583) (8.1266, -6.3747) (8.1266, -6.4395) knots 0 0 0 1 1 1
  spline S206 degree 2 poles (8.1266, -6.4395) (8.1266, -6.4762) (8.0744, -6.5362) (8.0347, -6.5362) knots 0 0 0 1 2 2 2
  spline S207 degree 2 poles (8.0347, -6.5362) (8.0212, -6.5362) (8.0096, -6.5323) knots 0 0 0 1 1 1
  spline S208 degree 2 poles (7.0518, -7.6302) (6.9377, -7.5375) (6.8498, -7.3606) (6.8498, -7.2359) knots 0 0 0 1 2 2 2
  spline S209 degree 2 poles (6.8498, -7.2359) (6.8498, -7.0233) (7.0296, -6.8889) knots 0 0 0 1 1 1
  spline S210 degree 2 poles (7.0296, -6.8889) (7.2113, -6.7507) (7.5051, -6.7507) knots 0 0 0 1 1 1
  spline S211 degree 2 poles (7.5051, -6.7507) (7.8298, -6.7507) (7.9999, -6.9063) knots 0 0 0 1 1 1
  spline S212 degree 2 poles (7.9999, -6.9063) (8.1362, -7.031) (8.1362, -7.2108) knots 0 0 0 1 1 1
  spline S213 degree 2 poles (8.1362, -7.2108) (8.1362, -7.3509) (8.0947, -7.4321) knots 0 0 0 1 1 1
  spline S214 degree 2 poles (8.0947, -7.4321) (8.0483, -7.522) (7.9332, -7.5848) knots 0 0 0 1 1 1
  spline S215 degree 2 poles (7.9332, -7.5848) (7.9091, -7.5984) (7.8869, -7.5984) knots 0 0 0 1 1 1
  spline S216 degree 2 poles (7.8869, -7.5984) (7.8482, -7.5984) (7.795, -7.5404) (7.795, -7.5046) knots 0 0 0 1 2 2 2
  spline S217 degree 2 poles (7.795, -7.5046) (7.795, -7.4543) (7.8492, -7.4253) knots 0 0 0 1 1 1
  spline S218 degree 2 poles (7.8492, -7.4253) (7.9052, -7.3925) (7.9294, -7.3364) knots 0 0 0 1 1 1
  spline S219 degree 2 poles (7.9294, -7.3364) (7.9497, -7.2939) (7.9497, -7.2098) knots 0 0 0 1 1 1
  spline S220 degree 2 poles (7.9497, -7.2098) (7.9497, -7.1006) (7.8521, -7.0252) knots 0 0 0 1 1 1
  spline S221 degree 2 poles (7.8521, -7.0252) (7.7341, -6.9324) (7.5051, -6.9324) knots 0 0 0 1 1 1
  spline S222 degree 2 poles (7.5051, -6.9324) (7.2944, -6.9324) (7.0363, -7.1074) (7.0363, -7.2388) knots 0 0 0 1 2 2 2
  spline S223 degree 2 poles (7.0363, -7.2388) (7.0363, -7.3809) (7.1716, -7.4882) knots 0 0 0 1 1 1
  spline S224 degree 2 poles (7.1716, -7.4882) (7.2045, -7.5152) (7.2045, -7.5568) knots 0 0 0 1 1 1
  spline S225 degree 2 poles (7.2045, -7.5568) (7.2045, -7.5926) (7.1475, -7.6525) (7.1098, -7.6525) knots 0 0 0 1 2 2 2
  spline S226 degree 2 poles (7.1098, -7.6525) (7.0788, -7.6525) (7.0518, -7.6302) knots 0 0 0 1 1 1
  spline S227 degree 2 poles (7.0518, -8.7582) (6.9377, -8.6654) (6.8498, -8.4885) (6.8498, -8.3638) knots 0 0 0 1 2 2 2
  spline S228 degree 2 poles (6.8498, -8.3638) (6.8498, -8.1512) (7.0296, -8.0169) knots 0 0 0 1 1 1
  spline S229 degree 2 poles (7.0296, -8.0169) (7.2113, -7.8786) (7.5051, -7.8786) knots 0 0 0 1 1 1
  spline S230 degree 2 poles (7.5051, -7.8786) (7.8298, -7.8786) (7.9999, -8.0342) knots 0 0 0 1 1 1
  spline S231 degree 2 poles (7.9999, -8.0342) (8.1362, -8.1589) (8.1362, -8.3387) knots 0 0 0 1 1 1
  spline S232 degree 2 poles (8.1362, -8.3387) (8.1362, -8.4788) (8.0947, -8.56) knots 0 0 0 1 1 1
  spline S233 degree 2 poles (8.0947, -8.56) (8.0483, -8.6499) (7.9332, -8.7127) knots 0 0 0 1 1 1
  spline S234 degree 2 poles (7.9332, -8.7127) (7.9091, -8.7263) (7.8869, -8.7263) knots 0 0 0 1 1 1
  spline S235 degree 2 poles (7.8869, -8.7263) (7.8482, -8.7263) (7.795, -8.6683) (7.795, -8.6325) knots 0 0 0 1 2 2 2
  spline S236 degree 2 poles (7.795, -8.6325) (7.795, -8.5823) (7.8492, -8.5533) knots 0 0 0 1 1 1
  spline S237 degree 2 poles (7.8492, -8.5533) (7.9052, -8.5204) (7.9294, -8.4643) knots 0 0 0 1 1 1
  spline S238 degree 2 poles (7.9294, -8.4643) (7.9497, -8.4218) (7.9497, -8.3377) knots 0 0 0 1 1 1
  spline S239 degree 2 poles (7.9497, -8.3377) (7.9497, -8.2285) (7.8521, -8.1531) knots 0 0 0 1 1 1
  spline S240 degree 2 poles (7.8521, -8.1531) (7.7341, -8.0603) (7.5051, -8.0603) knots 0 0 0 1 1 1
  spline S241 degree 2 poles (7.5051, -8.0603) (7.2944, -8.0603) (7.0363, -8.2353) (7.0363, -8.3667) knots 0 0 0 1 2 2 2
  spline S242 degree 2 poles (7.0363, -8.3667) (7.0363, -8.5088) (7.1716, -8.6161) knots 0 0 0 1 1 1
  spline S243 degree 2 poles (7.1716, -8.6161) (7.2045, -8.6432) (7.2045, -8.6847) knots 0 0 0 1 1 1
  spline S244 degree 2 poles (7.2045, -8.6847) (7.2045, -8.7205) (7.1475, -8.7804) (7.1098, -8.7804) knots 0 0 0 1 2 2 2
  spline S245 degree 2 poles (7.1098, -8.7804) (7.0788, -8.7804) (7.0518, -8.7582) knots 0 0 0 1 1 1
  spline S246 degree 2 poles (4.7805, -6.5738) (4.5244, -6.5738) (4.3987, -6.4327) knots 0 0 0 1 1 1
  spline S247 degree 2 poles (4.3987, -6.4327) (4.3098, -6.3332) (4.3098, -6.2008) knots 0 0 0 1 1 1
  spline S248 degree 2 poles (4.3098, -6.2008) (4.3098, -5.9756) (4.5427, -5.8248) knots 0 0 0 1 1 1
  spline S249 degree 2 poles (4.5427, -5.8248) (4.7022, -5.6943) (4.9438, -5.6943) knots 0 0 0 1 1 1
  spline S250 degree 2 poles (4.9438, -5.6943) (5.2386, -5.6943) (5.4145, -5.8306) knots 0 0 0 1 1 1
  spline S251 degree 2 poles (5.4145, -5.8306) (5.5962, -5.9688) (5.5962, -6.1805) knots 0 0 0 1 1 1
  spline S252 degree 2 poles (5.5962, -6.1805) (5.5962, -6.3284) (5.5189, -6.4269) knots 0 0 0 1 1 1
  spline S253 degree 2 poles (5.5189, -6.4269) (5.4967, -6.4724) (5.4019, -6.5352) knots 0 0 0 1 1 1
  spline S254 degree 2 poles (5.4019, -6.5352) (5.3768, -6.5526) (5.3469, -6.5526) knots 0 0 0 1 1 1
  spline S255 degree 2 poles (5.3469, -6.5526) (5.3101, -6.5526) (5.2589, -6.4965) (5.2589, -6.4608) knots 0 0 0 1 2 2 2
  spline S256 degree 2 poles (5.2589, -6.4608) (5.2589, -6.4134) (5.313, -6.3796) knots 0 0 0 1 1 1
  spline S257 degree 2 poles (5.313, -6.3796) (5.3614, -6.3399) (5.3768, -6.3158) knots 0 0 0 1 1 1
  spline S258 degree 2 poles (5.3768, -6.3158) (5.4097, -6.2665) (5.4097, -6.1805) knots 0 0 0 1 1 1
  spline S259 degree 2 poles (5.4097, -6.1805) (5.4097, -6.0452) (5.1555, -5.878) (4.9438, -5.878) knots 0 0 0 1 2 2 2
  spline S260 degree 2 poles (4.9438, -5.878) (4.7718, -5.878) (4.6403, -5.963) knots 0 0 0 1 1 1
  spline S261 degree 2 poles (4.6403, -5.963) (4.4963, -6.0558) (4.4963, -6.2008) knots 0 0 0 1 1 1
  spline S262 degree 2 poles (4.4963, -6.2008) (4.4963, -6.3235) (4.622, -6.3641) knots 0 0 0 1 1 1
  spline S263 degree 2 poles (4.622, -6.3641) (4.6829, -6.3854) (4.8046, -6.3854) knots 0 0 0 1 1 1
  line L56 (4.8046, -6.3854) -> (4.8046, -6.2394)
  spline S264 degree 2 poles (4.8046, -6.2394) (4.8046, -6.1457) (4.8984, -6.1457) knots 0 0 0 1 1 1
  spline S265 degree 2 poles (4.8984, -6.1457) (4.9912, -6.1457) (4.9912, -6.2394) knots 0 0 0 1 1 1
  line L57 (4.9912, -6.2394) -> (4.9912, -6.5738)
  line L58 (4.9912, -6.5738) -> (4.7805, -6.5738)
  spline S266 degree 2 poles (4.4103, -7.8187) (4.3166, -7.8187) (4.3166, -7.7404) knots 0 0 0 1 1 1
  spline S267 degree 2 poles (4.3166, -7.7404) (4.3166, -7.6853) (4.3678, -7.6496) knots 0 0 0 1 1 1
  line L59 (4.3678, -7.6496) -> (5.2492, -7.0745)
  line L60 (5.2492, -7.0745) -> (4.4122, -7.0745)
  spline S268 degree 2 poles (4.4122, -7.0745) (4.3166, -7.0745) (4.3166, -6.9827) knots 0 0 0 1 1 1
  spline S269 degree 2 poles (4.3166, -6.9827) (4.3166, -6.8909) (4.4122, -6.8909) knots 0 0 0 1 1 1
  line L61 (4.4122, -6.8909) -> (5.4996, -6.8909)
  spline S270 degree 2 poles (5.4996, -6.8909) (5.5885, -6.8909) (5.5885, -6.9759) knots 0 0 0 1 1 1
  spline S271 degree 2 poles (5.5885, -6.9759) (5.5885, -7.032) (5.5324, -7.0716) knots 0 0 0 1 1 1
  line L62 (5.5324, -7.0716) -> (4.6742, -7.6351)
  line L63 (4.6742, -7.6351) -> (5.4938, -7.6351)
  spline S272 degree 2 poles (5.4938, -7.6351) (5.5885, -7.6351) (5.5885, -7.7269) knots 0 0 0 1 1 1
  spline S273 degree 2 poles (5.5885, -7.7269) (5.5885, -7.8187) (5.4938, -7.8187) knots 0 0 0 1 1 1
  line L64 (5.4938, -7.8187) -> (4.4103, -7.8187)
  spline S274 degree 2 poles (4.997, -8.9408) (4.6577, -8.9408) (4.4799, -8.7611) knots 0 0 0 1 1 1
  spline S275 degree 2 poles (4.4799, -8.7611) (4.3349, -8.6161) (4.3349, -8.4054) knots 0 0 0 1 1 1
  line L65 (4.3349, -8.4054) -> (4.3349, -8.0681)
  line L66 (4.3349, -8.0681) -> (5.5846, -8.0681)
  line L67 (5.5846, -8.0681) -> (5.5846, -8.4044)
  spline S276 degree 2 poles (5.5846, -8.4044) (5.5846, -8.6122) (5.4474, -8.763) knots 0 0 0 1 1 1
  spline S277 degree 2 poles (5.4474, -8.763) (5.284, -8.9408) (4.997, -8.9408) knots 0 0 0 1 1 1
  spline S278 degree 2 poles (4.997, -8.7591) (5.1932, -8.7591) (5.3024, -8.6412) knots 0 0 0 1 1 1
  spline S279 degree 2 poles (5.3024, -8.6412) (5.3961, -8.5397) (5.3961, -8.4035) knots 0 0 0 1 1 1
  line L68 (5.3961, -8.4035) -> (5.3961, -8.2498)
  line L69 (5.3961, -8.2498) -> (4.5215, -8.2498)
  line L70 (4.5215, -8.2498) -> (4.5215, -8.4054)
  spline S280 degree 2 poles (4.5215, -8.4054) (4.5215, -8.5446) (4.6065, -8.6374) knots 0 0 0 1 1 1
  spline S281 degree 2 poles (4.6065, -8.6374) (4.7524, -8.7591) (4.997, -8.7591) knots 0 0 0 1 1 1
  point P0 (0, 0)
  point P1 (17.653, -5.588)
  point P2 (15.113, -5.588)
  point P3 (16.8609, -6.6209)
  point P4 (12.573, -5.588)
  point P5 (11.5583, -6.6209)
  point P6 (10.033, -5.588)
  point P7 (9.7619, -6.6209)
  point P8 (7.493, -5.588)
  point P9 (7.0131, -6.6209)
  point P10 (4.953, -5.588)
  point P11 (4.1243, -6.6209)
  point P12 (10.3041, -6.6209)
  dimension "d63" = 1.27
  constraints: 12 midpoint, 12 vertical alignment, 5 horizontal alignment, 12 other
  measures "d63" distance of A0.centre point (17.653, -5.588)
extrude "Extrusion9" add sketch "Sketch9" along normal blind 0.0254 contours S0 S1 S2 S3 S4 S5 S6 S7 S8 S9 S10 S11 S12 S13 S14 S15 S16 S17 S18 | S19 S20 S21 S22 S23 S24 S25 S26 S27 S28 S29 S30 S31 S32 S33 S34 S35 S36 S37 S38 S39 S40 S41 | S42 S43 S44 S45 S46 S47 S48 S49 S50 S51 S52 S53 S54 S55 S56 S57 S58 S59 S60 S61 S62 S63 S64 | S65 S66 S67 S68 S69 S70 S71 S72 S73 S74 S75 S76 S77 S78 S79 S80 S81 S82 S83 | S84 S85 S86 L24 L25 L26 S87 S88 L27 S89 S90 L28 L29 S91 S92 S93 L30 L31 | S94 S95 L32 L33 S96 S97 L34 L35 S98 S99 L36 S100 S101 L37 L38 S102 S103 L39 | S104 S105 S106 S107 S108 S109 S110 S111 | S120 S121 S122 S123 S124 S125 S126 S127 S128 S129 S130 S131 S132 S133 S134 S135 S136 S137 S138 S139 S140 S141 S142 | S143 S144 L40 S145 S146 L41 | S147 S148 L42 L43 S149 S150 L44 L45 S151 S152 L46 S153 S154 L47 L48 S155 S156 L49 | S157 S158 L50 S159 S160 L51 | S161 S162 S163 S164 S165 S166 S167 S168 S169 S170 S171 S172 S173 S174 S175 S176 S177 S178 S179 S180 S181 S182 S183 | S184 S185 S186 S187 S188 S189 S190 S191 | L52 S200 S201 L53 S202 S203 S204 L54 L55 S205 S206 S207 | S208 S209 S210 S211 S212 S213 S214 S215 S216 S217 S218 S219 S220 S221 S222 S223 S224 S225 S226 | S227 S228 S229 S230 S231 S232 S233 S234 S235 S236 S237 S238 S239 S240 S241 S242 S243 S244 S245 | S246 S247 S248 S249 S250 S251 S252 S253 S254 S255 S256 S257 S258 S259 S260 S261 S262 S263 L56 S264 S265 L57 L58 | S266 S267 L59 L60 S268 S269 L61 S270 S271 L62 L63 S272 S273 L64 | S274 S275 L65 L66 L67 S276 S277
equation "\"d9\" = d8"
equation "\"d10\" = d7"
equation "\"d40\" = d41"
body "Solid1"
